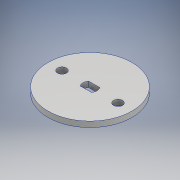
# Autodesk Inventor part: レスキューキット接続
Saved by Autodesk Inventor 2018 (Build 220112000, 112)
## iProperties
Created: 2018-08-22
Part Number: レスキューキット接続
Material: アルミニウム 6061
Document SubType Name: Modeling
Designer: shun2
Density: 2.7 g/cm^3
Appearance: アルミニウム - フラット
Author: shun2
Autodesk Inventor part; units mm, degrees
ref_plane "YZ Plane" through (0, 0, 0) normal (1, 0, 0) x (0, 1, 0)
ref_plane "XZ Plane" through (0, 0, 0) normal (0, 1, 0) x (-1, 0, 0)
ref_plane "XY Plane" through (0, 0, 0) normal (0, 0, 1) x (1, 0, 0)
sketch "スケッチ1" plane through (0, 0, 0) normal (0, 0, 1) x (1, 0, 0)
  line L0 (63, 56.862) -> (67, 56.862)
  line L1 (67, 53.862) -> (63, 53.862)
  arc A0 (67, 53.862) -> (67, 56.862) centre (65, 55.362) ccw
  arc A1 (63, 56.862) -> (63, 53.862) centre (65, 55.362) ccw
  circle A2 centre (65, 55.362) radius 15
  circle A3 centre (55, 55.362) radius 1.6
  circle A4 centre (75, 55.362) radius 1.6
  point P0 (0, 0)
  point P1 (65, 55.362)
  dimension "d1" = 30
  dimension "d7" = 3.2
  dimension "d8" = 3.2
  constraints: 5 centre point, 4 end point, 4 point on circle, 2 coincident, 1 horizontal, 1 parallel, 1 other
  measures "d1" diameter of A2
  measures "d7" diameter of A3
  measures "d8" diameter of A4
extrude "押し出し1" add sketch "スケッチ1" along normal blind 2
